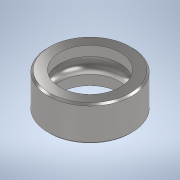
# Autodesk Inventor part: 6138k63_race
Saved by Autodesk Inventor 2020.1 (Build 241239000, 239)
## iProperties
Created: 2019-10-27
Part Number: 6138k63_race
Material: Stainless Steel, 440C
Document SubType Name: Modeling
Designer: agmle
Mass: 0.895595 g
Surface Area: 2.85754 cm^2
Volume: 0.115561 cm^3
Density: 7.75 g/cm^3
Appearance: Semi-Polished
Author: agmle
Autodesk Inventor part; units mm, degrees
ref_plane "YZ Plane" through (0, 0, 0) normal (1, 0, 0) x (0, 1, 0)
ref_plane "XZ Plane" through (0, 0, 0) normal (0, 1, 0) x (-1, 0, 0)
ref_plane "XY Plane" through (0, 0, 0) normal (0, 0, 1) x (1, 0, 0)
sketch "Sketch1" plane through (0, 0, 0) normal (0, 0, 1) x (1, 0, 0)
  line L0 (3.4192, 1.2639) -> (3.4192, 1.8852)
  line L1 (3.4192, 1.9844) -> (4.5641, 1.9844)
  line L2 (4.5641, 1.9844) -> (4.7625, 1.7859)
  line L3 (4.7625, 1.7859) -> (4.7625, 0)
  line L4 (0, 0) -> (4.7625, 0) construction
  line L5 (3.4192, 1.9844) -> (3.4192, 1.8852)
  line L6 (3.4192, 1.2639) -> (3.4192, 0.8819)
  arc A0 (4.0901, 0) -> (3.4192, 0.8819) centre (3.175, 0) ccw
  line L7 (3.4192, -1.2639) -> (3.4192, -1.8852)
  line L8 (3.4192, -1.9844) -> (4.5641, -1.9844)
  line L9 (4.5641, -1.9844) -> (4.7625, -1.7859)
  line L10 (4.7625, -1.7859) -> (4.7625, 0)
  line L11 (3.4192, -1.9844) -> (3.4192, -1.8852)
  line L12 (3.4192, -1.2639) -> (3.4192, -0.8819)
  arc A1 (3.4192, -0.8819) -> (4.0901, 0) centre (3.175, 0) ccw
  line L13 (0, -2.7781) -> (0, 2.7781) projected
  dimension "d0" = 0.2806
  dimension "d1" = 1.1448
  dimension "d2" = 0.9151
  dimension "d3" = 0.0992
  dimension "d4" = 0
  dimension "d5" = 1.9844
  dimension "d6" = 1.3433
  dimension "d7" = 4.7625
  dimension "d8" = 0.2442
  constraints: 26 end point, 8 symmetric about line, 6 point on line, 4 point on circle, 2 centre point, 2 coincident, 2 vertical, 1 horizontal, 1 parallel, 1 perpendicular, 5 other
  measures "d0" distance of L1.end L2.end
  measures "d1" distance of L1.start L1.end
  measures "d2" radius of A0
  measures "d3" distance of L1.start L5.end
  measures "d4" distance of L5.end L0.end
  measures "d5" distance between parallel lines of L4 L1
  measures "d6" distance between parallel lines of L3 L5
  measures "d7" distance from line of L4.start L3
  measures "d8" distance from line of A0.centre L6
revolve "Revolution1" add sketch "Sketch1" angle 360 about axis through (0, -10, 0) along (0, 1, 0)
body "Solid1"
